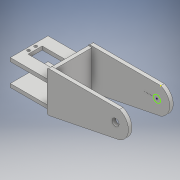
# Autodesk Inventor part: Femur
Saved by Autodesk Inventor 2018 (Build 220112000, 112)
## iProperties
Created: 2020-03-07
Part Number: Femur
Material: Generic
Document SubType Name: Modeling
Designer: GonzaloDiaz
Density: 1 g/cm^3
Appearance: Default
Author: GonzaloDiaz
Autodesk Inventor part; units mm, degrees
ref_plane "YZ Plane" through (0, 0, 0) normal (1, 0, 0) x (0, 1, 0)
ref_plane "XZ Plane" through (0, 0, 0) normal (0, 1, 0) x (-1, 0, 0)
ref_plane "XY Plane" through (0, 0, 0) normal (0, 0, 1) x (1, 0, 0)
sketch "servo_frontal" plane through (0, 0, 0) normal (0, 0, 1) x (1, 0, 0)
  line L0 (-55.8999, 17.5383) -> (-55.8999, 37.5416)
  line L1 (-1.4999, 37.5416) -> (-1.4999, 17.5383)
  line L2 (-55.8999, 37.5416) -> (-1.4999, 37.5416)
  line L3 (-1.4999, 37.5416) -> (-1.4999, 17.5383)
  line L4 (-1.4999, 17.5383) -> (-55.8999, 17.5383)
  line L5 (-55.8999, 17.5383) -> (-55.8999, 37.5416)
  circle A0 centre (-52.7956, 32.5408) radius 2
  circle A1 centre (-52.7956, 32.5408) radius 2
  circle A2 centre (-52.7956, 22.5391) radius 2
  circle A3 centre (-52.7956, 22.5391) radius 2
  circle A4 centre (-4.6894, 22.5391) radius 2
  circle A5 centre (-4.6894, 22.5391) radius 2
  circle A6 centre (-4.6894, 32.5408) radius 2
  circle A7 centre (-4.6894, 32.5408) radius 2
  line L6 (-8.6999, 17.5383) -> (-48.6999, 17.5383)
  line L7 (-8.6999, 17.5383) -> (-48.6999, 17.5383)
  line L8 (-48.6999, 17.5383) -> (-48.6999, 37.5416)
  line L9 (-48.6999, 37.5416) -> (-8.6999, 37.5416)
  line L10 (-8.6999, 37.5416) -> (-8.6999, 17.5383)
  point P0 (-29.1054, 26.9516)
ref_plane "Work Plane10" through (0, -30, 0) normal (0, -1, 0) x (1, 0, 0)
sketch "Sketch4" plane through (0, -30, 0) normal (0, -1, 0) x (1, 0, 0)
  line L0 (-102, -2) -> (-102, -55.2)
  line L1 (-99.607, -57.161) -> (0, -37.1993)
  line L2 (0, -37.1993) -> (0, 0) construction
  line L3 (-100, 0) -> (0, 0)
  arc A0 (0, -37.1993) -> (0, 0) centre (-7.352, -18.5997) ccw
  arc A1 (-102, -55.2) -> (-99.607, -57.161) centre (-100, -55.2) ccw
  arc A2 (-100, 0) -> (-102, -2) centre (-100, -2) ccw
  point P0 (-102, 0)
  point P1 (-102, -57.6406)
  dimension "d4" = 20
  dimension "d5" = 2
  dimension "d6" = 2
  dimension "d12" = 100
  dimension "d55" = 53.2
  constraints: 8 end point, 6 point on circle, 4 point on line, 4 tangent, 3 centre point, 1 coincident, 1 horizontal, 1 perpendicular, 1 vertical
  measures "d4" radius of A0
  measures "d5" radius of A1
  measures "d6" radius of A2
  measures "d12" distance of L3.start L2.end
  measures "d55" distance of L0.start L0.end
extrude "Extrusion1" add sketch "Sketch4" along normal blind 5
ref_plane "Work Plane3" through (0, 23.2, 0) normal (0, 1, 0) x (1, 0, 0)
ref_plane "Work Plane4" through (0, -3.4, 0) normal (0, 1, 0) x (1, 0, 0)
mirror "Mirror3" about plane through (0, -3.4, 0) normal (0, 1, 0) of "Extrusion1"
sketch "Sketch9" plane through (0, -35, 0) normal (0, -1, 0) x (1, 0, 0)
  circle A0 centre (-5.4629, -18.5) radius 5
  arc A1 (0, -37.1993) -> (0, 0) centre (-7.352, -18.5997) ccw projected
  line L0 (0, -37) -> (0, 0)
  dimension "d20" = 10
  dimension "d21" = 18.5
  dimension "d22" = 37
  constraints: 2 end point, 1 centre point, 1 vertical
  measures "d20" diameter of A0
  measures "d21" vertical distance of L0.end A0.centre
  measures "d22" distance of L0.start L0.end
extrude "Extrusion2" cut sketch "Sketch9" against normal blind 5
sketch "Sketch11" plane through (-102, -30, -55.2) normal (-1, 0, 0) x (0, 0, 1)
  line L0 (53.2, 53.2) -> (53.2, 58.2) projected
  line L1 (0, 0) -> (53.2, 0) projected
  line L2 (53.2, 53.2) -> (0, 53.2)
  line L3 (0, 53.2) -> (0, 0)
  line L4 (0, 0) -> (53.2, 0)
  line L5 (53.2, 0) -> (53.2, 53.2)
  constraints: 8 end point, 2 parallel, 1 horizontal, 1 perpendicular
sketch "Sketch12" plane through (-100, 23.2, 0) normal (0, -1, 0) x (1, 0, 0)
  circle A0 centre (94.5371, -18.5) radius 5 projected
  circle A1 centre (94.5371, -18.5) radius 5
  point P0 (100, 0)
  constraints: 1 centre point, 1 coincident
sketch "Sketch13" plane through (-100, 23.2, 0) normal (0, -1, 0) x (1, 0, 0)
  circle A0 centre (94.5207, -18.4668) radius 1.125
  circle A1 centre (89.5207, -18.4668) radius 0.3
  circle A2 centre (87.5207, -18.4668) radius 0.3
  circle A3 centre (85.5207, -18.4668) radius 0.3
  circle A4 centre (83.5207, -18.4668) radius 0.3
  circle A5 centre (81.5207, -18.4668) radius 0.3
  circle A6 centre (79.5207, -18.4668) radius 0.3
  circle A7 centre (77.5063, -18.4668) radius 0.3144
  point P0 (0, 0)
  constraints: 8 centre point
extrude "Extrusion5" cut sketch "Sketch13" against normal blind 5
extrude "Extrusion6" add sketch "Sketch11" against normal blind 5
sketch "Sketch18" plane through (-102, -35, -55.2) normal (-1, 0, 0) x (0, 0, 1)
  line L0 (0, 58.2) -> (0, 63.2) projected
  line L1 (18.0007, 5) -> (-1.961, 5) projected
  line L2 (0, 58.2) -> (5, 58.2)
  line L3 (5, 58.2) -> (5, 5)
  line L4 (5, 5) -> (0, 5)
  line L5 (0, 5) -> (0, 58.2)
  line L6 (55.2, 58.2) -> (18.0007, 58.2) projected
  line L7 (55.2, 5) -> (18.0007, 5) projected
  line L8 (31.6, 58.2) -> (36.6, 58.2)
  line L9 (36.6, 58.2) -> (36.6, 5)
  line L10 (36.6, 5) -> (31.6, 5)
  line L11 (31.6, 5) -> (31.6, 58.2)
  point P0 (55.2, 35)
  dimension "d58" = 5
  dimension "d59" = 5
  dimension "d60" = 26.6
  constraints: 16 end point, 4 parallel, 3 point on line, 2 horizontal, 2 perpendicular
  measures "d58" distance of L3.end L4.end
  measures "d59" distance of L9.end L10.end
  measures "d60" distance between parallel lines of L11 L3
extrude "Extrusion7" add sketch "Sketch18" along normal blind 57
sketch "Sketch21" plane through (-102, -30, -18.6) normal (0, 0, 1) x (1, 0, 0)
  line L0 (0, 0) -> (-57, 0) projected
  line L1 (-57, 0) -> (-57, 53.2) projected
  line L2 (-55.8999, 16.6) -> (-55.8999, 36.6033)
  line L3 (-1.4999, 36.6033) -> (-1.4999, 16.6)
  line L4 (-55.8999, 36.6033) -> (-1.4999, 36.6033)
  line L5 (-1.4999, 36.6033) -> (-1.4999, 16.6)
  line L6 (-1.4999, 16.6) -> (-55.8999, 16.6)
  line L7 (-55.8999, 16.6) -> (-55.8999, 36.6033)
  circle A0 centre (-52.7956, 31.6025) radius 2
  circle A1 centre (-52.7956, 31.6025) radius 2
  circle A2 centre (-52.7956, 21.6008) radius 2
  circle A3 centre (-52.7956, 21.6008) radius 2
  circle A4 centre (-4.6894, 21.6008) radius 2
  circle A5 centre (-4.6894, 21.6008) radius 2
  circle A6 centre (-4.6894, 31.6025) radius 2
  circle A7 centre (-4.6894, 31.6025) radius 2
  line L8 (-8.6999, 16.6) -> (-48.6999, 16.6)
  line L9 (-8.6999, 16.6) -> (-48.6999, 16.6)
  line L10 (-48.6999, 16.6) -> (-48.6999, 36.6033)
  line L11 (-48.6999, 36.6033) -> (-8.6999, 36.6033)
  line L12 (-8.6999, 36.6033) -> (-8.6999, 16.6)
  point P0 (102, 30)
  dimension "d73" = 16.6
  dimension "d74" = 1.1001
extrude "Extrusion8" cut sketch "Sketch21" against normal blind 5 contours L10 L4 L12 L6 | A0 | A2 | A4 | A6
body "Solid1"
